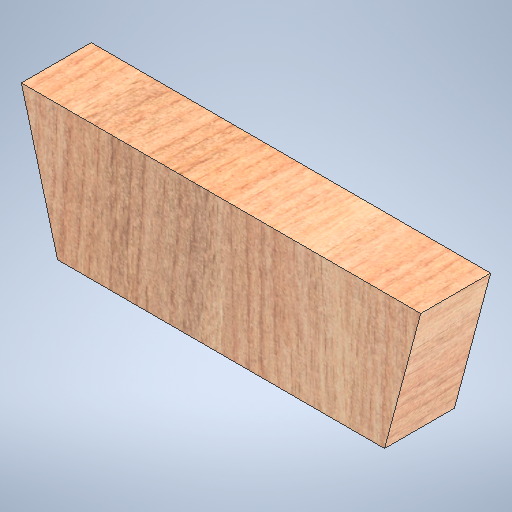
# Autodesk Inventor part: Corner Stone
Saved by Autodesk Inventor 2025 (Build 290162000, 162)
## iProperties
Created: 2024-07-01
Part Number: Corner Stone
Material: Generic
Document SubType Name: Modeling
Designer: Cupri
Density: 1 g/cm^3
Appearance: Default
Author: Cupri
Autodesk Inventor part; units mm, degrees
ref_plane "YZ Plane" through (0, 0, 0) normal (1, 0, 0) x (0, 1, 0)
ref_plane "XZ Plane" through (0, 0, 0) normal (0, 1, 0) x (-1, 0, 0)
ref_plane "XY Plane" through (0, 0, 0) normal (0, 0, 1) x (1, 0, 0)
sketch "Sketch1" plane through (0, 0, 0) normal (0, 0, 1) x (1, 0, 0)
  line L0 (0, 0) -> (290.2712, 0)
  line L1 (290.2712, 0) -> (263.9752, -98.1381)
  line L2 (0, 0) -> (26.296, -98.1381)
  line L3 (26.296, -98.1381) -> (263.9752, -98.1381)
  dimension "d0" = 290.2712
  dimension "d1" = 101.6
  dimension "d2" = 75
  dimension "d3" = 101.6
  dimension "d4" = 75
  constraints: 8 end point, 1 horizontal
  measures "d0" distance of L0.start L0.end
  measures "d1" distance of L0.end L1.end
  measures "d2" angle of L1 L0
  measures "d3" distance of L0.start L2.end
  measures "d4" angle of L0 L2
extrude "Extrusion1" add sketch "Sketch1" along normal blind 50.8
body "Solid1"
